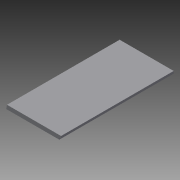
# Autodesk Inventor part: regalboden
Saved by Autodesk Inventor 2013 (Build 170138000, 138)
## iProperties
Created: 2014-03-31
Part Number: regalboden
Material: Generic
Document SubType Name: Modeling
Designer: hhanff
Density: 1 g/cm^3
Author: hhanff
Autodesk Inventor part; units mm, degrees
ref_plane "YZ Plane" through (0, 0, 0) normal (1, 0, 0) x (0, 1, 0)
ref_plane "XZ Plane" through (0, 0, 0) normal (0, 1, 0) x (-1, 0, 0)
ref_plane "XY Plane" through (0, 0, 0) normal (0, 0, 1) x (1, 0, 0)
sketch "Sketch1" plane through (0, 0, 0) normal (0, 0, 1) x (1, 0, 0)
  line L0 (0, 0) -> (243.149, 0)
  line L1 (243.149, 0) -> (243.149, 500)
  line L2 (243.149, 500) -> (0, 500)
  line L3 (0, 500) -> (0, 0)
  dimension "d0" = 243.149
  dimension "d1" = 500
  constraints: 8 end point, 2 parallel, 1 horizontal, 1 perpendicular
  measures "d0" distance of L1.end L2.end
  measures "d1" distance of L2.end L0.start
extrude "Extrusion1" add sketch "Sketch1" along normal blind 18
sketch "Sketch2" plane through (0, 0, 0) normal (0, 0, -1) x (-1, 0, 0)
  line L0 (0, 0) -> (-243.149, 0) projected
  line L1 (-243.149, 500) -> (-235.149, 500)
  line L2 (-235.149, 500) -> (-235.149, 0)
  line L3 (-235.149, 0) -> (-243.149, 0)
  line L4 (-243.149, 0) -> (-243.149, 500)
  dimension "d4" = 8
  constraints: 8 end point, 2 parallel, 1 horizontal, 1 perpendicular, 1 point on line
  measures "d4" distance of L2.end L3.end
extrude "Extrusion2" cut sketch "Sketch2" against normal blind 8
sketch "Sketch4" plane through (0, 500, 18) normal (0, 1, 0) x (1, 0, 0)
  line L0 (0, 18) -> (0, 0) projected
  line L1 (243.149, 0) -> (0, 0) projected
  line L2 (0, 0) -> (3.1489, 0)
  line L3 (0, 18) -> (0, 0)
  line L4 (3.1489, 0) -> (0, 18)
  dimension "d11" = 9.923
  constraints: 6 end point, 1 collinear, 1 point on line
  measures "d11" angle of L3 L4
extrude "Extrusion4" cut sketch "Sketch4" against normal up to next
body "Solid1"
